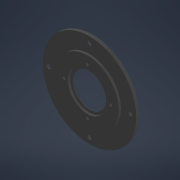
# Autodesk Inventor part: Фланец
Saved by Autodesk Inventor 2022 (Build 260153070, 153G)
## iProperties
Created: 2021-11-19
Part Number: Фланец
Material: Типовые
Document SubType Name: Modeling
Designer: kalugin_a
Density: 1 g/cm^3
Appearance: По умолчанию
Author: kalugin_a
Autodesk Inventor part; units mm, degrees
ref_plane "YZ Plane" through (0, 0, 0) normal (1, 0, 0) x (0, 1, 0)
ref_plane "XZ Plane" through (0, 0, 0) normal (0, 1, 0) x (-1, 0, 0)
ref_plane "XY Plane" through (0, 0, 0) normal (0, 0, 1) x (1, 0, 0)
sketch "Эскиз1" plane through (0, 0, 0) normal (0, 0, 1) x (1, 0, 0)
  circle A0 centre (0, 0) radius 52
  circle A1 centre (0, 0) radius 18.5
  point P0 (-24.7306, 0)
  point P1 (-47.5925, 0)
  dimension "d0" = 104
  dimension "d1" = 37
  constraints: 5 coincident, 2 centre point
  measures "d0" diameter of A0
  measures "d1" diameter of A1
extrude "Выдавливание1" add sketch "Эскиз1" against normal blind 3.5
sketch "Эскиз2" plane through (0, 0, 0) normal (0, 0, 1) x (1, 0, 0)
  circle A0 centre (0, 0) radius 35
  circle A1 centre (0, 0) radius 21.5934
  circle A2 centre (0, 0) radius 42.5 construction
  line L0 (0, 0) -> (30.052, -30.052) construction
  line L1 (0, 0) -> (42.5, 0) construction
  dimension "d41" = 85
  dimension "d4" = 70
  dimension "d42" = 45
  constraints: 4 end point, 3 coincident, 2 centre point, 1 equal length, 1 horizontal, 3 other
  measures "d4" diameter of A0
  measures "d42" angle of L0 L1
extrude "Выдавливание2" add sketch "Эскиз2" along normal blind 2.5
chamfer "Фаска1" distance 3 angle 45 1 edges at (-18.5, 0, -3.5)
sketch "Эскиз3" plane through (0, 0, -3.5) normal (0, 0, -1) x (-1, 0, 0)
  point P0 (0, 0)
  point P1 (46.0134, -0.1204)
hole "Отверстие1" at (-46.0134, -0.1204, -3.5) direction (0, 0, -1) diameter 4.5 end through all countersink diameter 8.3 countersink angle 90
sketch "Эскиз4" plane through (0, 0, -3.5) normal (0, 0, -1) x (-1, 0, 0)
  point P0 (0, 0)
  point P1 (45.4793, 0)
  point P2 (0, 45.4793)
  point P3 (-45.4793, 0)
  point P4 (0, -45.4793)
  dimension "d26" = 360
  constraints: 5 other
hole "Отверстие2" at (-45.4793, 0, -3.5) direction (0, 0, 1) diameter 4.5 end through all start extended yes countersink diameter 8.3 countersink angle 90
pattern_circular "Круговой массив1" count 4 over 360 about axis through (0, 0, -2) along (0, 0, -1) of "Отверстие2"
sketch "Эскиз5" plane through (0, 0, -3.5) normal (0, 0, -1) x (-1, 0, 0)
  point P0 (0, 0)
  point P1 (26.0216, -0.1377)
hole "Отверстие3" at (-26.0216, -0.1377, -3.5) direction (0, 0, 1) diameter 3 end through all start extended yes countersink diameter 6.4 countersink angle 90
pattern_circular "Круговой массив2" count 4 over 360 about axis through (0, 0, -2) along (0, 0, -1) of "Отверстие3"
